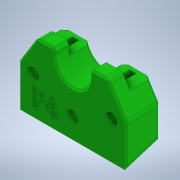
# Autodesk Inventor part: Y-Rod Holder
Saved by Autodesk Inventor 2020 (Build 240168000, 168)
## iProperties
Created: 2019-06-18
Part Number: Y-Rod Holder
Material: ABS Plastic
Document SubType Name: Modeling
Designer: pepd9
Density: 1.06 g/cm^3
Appearance: Dark Green
Author: pepd9
Autodesk Inventor part; units mm, degrees
ref_plane "YZ Plane" through (0, 0, 0) normal (1, 0, 0) x (0, 1, 0)
ref_plane "XZ Plane" through (0, 0, 0) normal (0, 1, 0) x (-1, 0, 0)
ref_plane "XY Plane" through (0, 0, 0) normal (0, 0, 1) x (1, 0, 0)
sketch "Sketch1" plane through (0, 0, 0) normal (0, 0, 1) x (1, 0, 0)
  circle A0 centre (0, 0) radius 5
  line L0 (-8, 0) -> (8, 0)
  line L1 (8, 0) -> (8, -12)
  line L2 (8, -12) -> (-8, -12)
  line L3 (-8, -12) -> (-8, 0)
  point P0 (5, 0)
  point P1 (-5, 0)
  dimension "d0" = 10
  dimension "d1" = 8
  dimension "d2" = 8
  dimension "d3" = 12
  constraints: 8 end point, 2 parallel, 1 centre point, 1 coincident, 1 horizontal, 1 perpendicular
  measures "d0" diameter of A0
  measures "d1" distance from line of L1 point (0, 0)
  measures "d2" distance of point (0, 0) L0.start
  measures "d3" distance from line of point (0, 0) L2
extrude "Extrusion1" add sketch "Sketch1" along normal blind 6 contours L0 L1 L2 L3 A0
sketch "Sketch2" plane through (0, 0, 6) normal (0, 0, 1) x (1, 0, 0)
  circle A0 centre (0, 0) radius 5 projected
  line L0 (-15, -18) -> (15, -18)
  line L1 (15, -18) -> (15, 2)
  line L2 (15, 2) -> (-15, 2)
  line L3 (-15, 2) -> (-15, -18)
  point P0 (0, 0)
  point P1 (4.5826, 2)
  point P2 (-4.5826, 2)
  dimension "d6" = 2
  dimension "d7" = 20
  dimension "d8" = 30
  dimension "d9" = 15
  constraints: 8 end point, 2 parallel, 1 horizontal, 1 perpendicular
  measures "d6" distance from line of L2 point (0, 0)
  measures "d7" distance between parallel lines of L2 L0
  measures "d8" distance of L1.end L2.end
  measures "d9" distance from line of L1 point (0, 0)
extrude "Extrusion2" add sketch "Sketch2" against normal blind 10 contours A0 L2 L1 L0 L3
chamfer "Chamfer1" distance 1 angle 45 2 edges at (-4.5826, 2, 1) (4.5826, 2, 1)
sketch "Sketch3" plane through (-15, 2, 6) normal (0, 1, 0) x (1, 0, 0)
  line L0 (9.1674, 5.5) -> (7.3674, 5.5)
  line L1 (7.3674, 5.5) -> (7.3674, 9)
  line L2 (7.3674, 9) -> (9.1674, 9)
  line L3 (9.1674, 9) -> (9.1674, 5.5)
  line L4 (9.1674, 5.5) -> (7.3674, 9) construction
  line L5 (7.3674, 5.5) -> (9.1674, 9) construction
  line L6 (0, 10) -> (9.4174, 10) projected
  line L7 (9.4174, 10) -> (9.4174, 0) projected
  point P0 (15, 6)
  point P1 (8.2674, 7.25)
  dimension "d15" = 1.8
  dimension "d16" = 3.5
  dimension "d17" = 1
  dimension "d18" = 0.25
  constraints: 12 end point, 2 midpoint, 2 parallel, 1 horizontal, 1 perpendicular
  measures "d15" distance of L1.end L2.end
  measures "d16" distance of L0.end L1.end
  measures "d17" distance between parallel lines of L6 L2
  measures "d18" distance between parallel lines of L3 L7
ref_plane "Work Plane1" through (0, 0, -3) normal (0, 0, -1) x (-1, 0, 0)
sketch "Sketch4" plane through (0, 0, -3) normal (0, 0, -1) x (-1, 0, 0)
  line L0 (15, 2) -> (5.5826, 2) projected
  line L1 (5.8326, 2) -> (7.2498, -1.8938)
  arc A0 (4.3864, -5.3999) -> (7.3385, -2.9339) centre (4.3864, -2.3999) ccw
  line L2 (4.3864, -5.3999) -> (0, -5.3999)
  arc A1 (-4.8889, 1.0481) -> (4.8889, 1.0481) centre (0, 0) ccw projected
  line L3 (0, 0) -> (0, 3.0326)
  line L4 (-5.8326, 2) -> (-7.2498, -1.8938)
  arc A2 (-7.3385, -2.9339) -> (-4.3864, -5.3999) centre (-4.3864, -2.3999) ccw
  line L5 (-4.3864, -5.3999) -> (0, -5.3999)
  arc A3 (7.3385, -2.9339) -> (7.2498, -1.8938) centre (5.3704, -2.5779) ccw
  arc A4 (-7.2498, -1.8938) -> (-7.3385, -2.9339) centre (-5.3704, -2.5779) ccw
  point P0 (0, 0)
  point P1 (7.3831, -2.2602)
  point P2 (-7.3831, -2.2602)
  point P3 (7.3831, -2.2602)
  point P4 (5.8326, 2)
  point P5 (-7.3831, -2.2602)
  dimension "d20" = 6
  dimension "d24" = 70
  dimension "d25" = 2
  constraints: 12 point on circle, 10 end point, 5 symmetric about line, 5 tangent, 4 centre point, 4 point on line, 1 equal radius, 1 horizontal, 1 vertical, 1 other
  measures "d20" diameter of A0
  measures "d24" angle of L0 L1
  measures "d25" radius of A3
sweep "Sweep1" cut profiles "Sketch3" path "Sketch4" path curves L1 A3 A0 L2 L5 A2 A4 L4
sketch "Sketch5" plane through (0, 0, 6) normal (0, 0, 1) x (1, 0, 0)
  line L0 (5.8326, 2) -> (7.6326, 2) projected
  line L1 (7.2498, -1.8938) -> (5.8326, 2) projected
  arc A0 (7.3385, -2.9339) -> (7.2498, -1.8938) centre (5.3704, -2.5779) ccw projected
  arc A1 (4.3864, -5.3999) -> (7.3385, -2.9339) centre (4.3864, -2.3999) ccw projected
  line L2 (-4.3864, -5.3999) -> (4.3864, -5.3999) projected
  arc A2 (-7.3385, -2.9339) -> (-4.3864, -5.3999) centre (-4.3864, -2.3999) ccw projected
  arc A3 (-7.2498, -1.8938) -> (-7.3385, -2.9339) centre (-5.3704, -2.5779) ccw projected
  line L3 (-5.8326, 2) -> (-7.2498, -1.8938) projected
  line L4 (-7.6326, 2) -> (-5.8326, 2) projected
  line L5 (-7.6326, 2) -> (-9.0498, -1.8938) projected
  arc A4 (-9.0498, -1.8938) -> (-8.8933, -3.8408) centre (-5.3704, -2.5779) ccw projected
  arc A5 (-8.8933, -3.8408) -> (-3.7708, -7.0913) centre (-4.3864, -2.3999) ccw projected
  line L6 (-3.7708, -7.0913) -> (5.002, -7.0913) projected
  arc A6 (5.002, -7.0913) -> (9.1125, -2.6292) centre (4.3864, -2.3999) ccw projected
  arc A7 (9.1125, -2.6292) -> (8.6287, -0.7368) centre (5.3704, -2.5779) ccw projected
  line L7 (8.6287, -0.7368) -> (7.6326, 2) projected
  line L8 (-9.4123, -4.3413) -> (-7.8246, -7.0913)
  line L9 (-7.8246, -7.0913) -> (-9.4123, -9.8413)
  line L10 (-9.4123, -9.8413) -> (-12.5877, -9.8413)
  line L11 (-12.5877, -9.8413) -> (-14.1754, -7.0913)
  line L12 (-14.1754, -7.0913) -> (-12.5877, -4.3413)
  line L13 (-12.5877, -4.3413) -> (-9.4123, -4.3413)
  line L14 (1.5877, -9.25) -> (3.1754, -12)
  line L15 (3.1754, -12) -> (1.5877, -14.75)
  line L16 (1.5877, -14.75) -> (-1.5877, -14.75)
  line L17 (-1.5877, -14.75) -> (-3.1754, -12)
  line L18 (-3.1754, -12) -> (-1.5877, -9.25)
  line L19 (-1.5877, -9.25) -> (1.5877, -9.25)
  line L20 (0, 0) -> (0, 7.1717)
  line L21 (9.4123, -4.3413) -> (7.8246, -7.0913)
  line L22 (7.8246, -7.0913) -> (9.4123, -9.8413)
  line L23 (9.4123, -9.8413) -> (12.5877, -9.8413)
  line L24 (12.5877, -9.8413) -> (14.1754, -7.0913)
  line L25 (14.1754, -7.0913) -> (12.5877, -4.3413)
  line L26 (12.5877, -4.3413) -> (9.4123, -4.3413)
  point P0 (0, -12)
  point P1 (-11, -7.0913)
  point P2 (-11, -7.0913)
  point P3 (0, -12)
  point P4 (11, -7.0913)
  dimension "d28" = 5.5
  dimension "d29" = 5.5
  dimension "d31" = 11
  dimension "d32" = 12
  constraints: 38 end point, 7 symmetric about line, 2 coincident, 1 vertical, 1 vertical alignment, 26 other
  measures "d28" distance between parallel lines of L13 L10
  measures "d29" distance between parallel lines of L16 L19
  measures "d31" horizontal distance of L20.start point (-11, -7.091)
  measures "d32" distance of L20.start point (0, -12)
sketch "Sketch6" plane through (0, 0, -4) normal (0, 0, -1) x (-1, 0, 0)
  line L0 (-9.4123, -4.3413) -> (-7.8246, -7.0913)
  line L1 (-7.8246, -7.0913) -> (-9.4123, -9.8413)
  line L2 (-9.4123, -9.8413) -> (-12.5877, -9.8413)
  line L3 (-12.5877, -9.8413) -> (-14.1754, -7.0913)
  line L4 (-14.1754, -7.0913) -> (-12.5877, -4.3413)
  line L5 (-12.5877, -4.3413) -> (-9.4123, -4.3413)
  line L6 (1.5877, -9.25) -> (3.1754, -12)
  line L7 (3.1754, -12) -> (1.5877, -14.75)
  line L8 (1.5877, -14.75) -> (-1.5877, -14.75)
  line L9 (-1.5877, -14.75) -> (-3.1754, -12)
  line L10 (-3.1754, -12) -> (-1.5877, -9.25)
  line L11 (-1.5877, -9.25) -> (1.5877, -9.25)
  line L12 (12.5877, -4.3413) -> (14.1754, -7.0913)
  line L13 (14.1754, -7.0913) -> (12.5877, -9.8413)
  line L14 (12.5877, -9.8413) -> (9.4123, -9.8413)
  line L15 (9.4123, -9.8413) -> (7.8246, -7.0913)
  line L16 (7.8246, -7.0913) -> (9.4123, -4.3413)
  line L17 (9.4123, -4.3413) -> (12.5877, -4.3413)
  point P0 (0, 0)
  point P1 (-11, -7.0913)
  point P2 (0, -12)
  point P3 (11, -7.0913)
  point P4 (-11, -7.0913)
  point P5 (0, -12)
  point P6 (11, -7.0913)
  point P7 (11, -4.3413)
  dimension "d33" = 5.5
  dimension "d34" = 5.5
  dimension "d35" = 5.5
  constraints: 36 end point, 3 coincident, 1 midpoint, 1 point on line, 39 other
  measures "d33" distance between parallel lines of L5 L2
  measures "d34" distance between parallel lines of L11 L8
  measures "d35" distance between parallel lines of L17 L14
extrude "Extrusion3" cut sketch "Sketch6" against normal blind 5
hole "Hole1" at (0, -12, 6) at (-11, -7.0913, 6) at (11, -7.0913, 6) direction (0, 0, -1) diameter 3.2 end through all
chamfer "Chamfer2" distance 8 distance2 5 1 edges at (-15, 2, 1) measured on face at (-15, 1.5, 1)
chamfer "Chamfer3" distance 5 distance2 8 1 edges at (15, 2, 1) measured on face at (14.5, 2, 1)
chamfer "Chamfer4" distance 0.25 distance2 4.5 1 edges at (11, -4.3413, -4) measured on face at (11, -3.8413, -4)
chamfer "Chamfer5" distance 0.25 distance2 4.5 2 edges at (12.5155, -4.2163, -4) (13.3816, -5.7163, -4) measured on face at (12.9486, -3.9663, -4) measured on face at (13.8146, -5.4663, -4)
chamfer "Chamfer6" distance 0.25 distance2 4.5 2 edges at (14.2476, -6.9663, -4) (13.3816, -8.4663, -4) measured on face at (14.6806, -7.2163, -4) measured on face at (13.8146, -8.7163, -4)
chamfer "Chamfer7" distance 0.25 distance2 4.5 2 edges at (12.7321, -9.8413, -4) (11, -9.8413, -4) measured on face at (11, -10.3413, -4) measured on face at (12.7321, -10.3413, -4)
chamfer "Chamfer8" distance 0.25 distance2 4.5 2 edges at (9.4845, -9.9663, -4) (8.6184, -8.4663, -4) measured on face at (9.0514, -10.2163, -4) measured on face at (8.1854, -8.7163, -4)
chamfer "Chamfer9" distance 0.25 distance2 4.5 3 edges at (7.7524, -7.2163, -4) (8.6184, -5.7163, -4) (9.4845, -4.2163, -4) measured on face at (7.3194, -6.9663, -4) measured on face at (9.0514, -3.9663, -4) measured on face at (8.1854, -5.4663, -4)
chamfer "Chamfer10" distance 0.25 distance2 4.5 1 edges at (0, -9.25, -4) measured on face at (0, -8.75, -4)
chamfer "Chamfer11" distance 0.25 distance2 4.5 2 edges at (1.5155, -9.125, -4) (2.3816, -10.625, -4) measured on face at (1.9486, -8.875, -4) measured on face at (2.8146, -10.375, -4)
chamfer "Chamfer12" distance 0.25 distance2 4.5 2 edges at (3.2476, -11.875, -4) (2.3816, -13.375, -4) measured on face at (2.8146, -13.625, -4) measured on face at (3.6806, -12.125, -4)
chamfer "Chamfer13" distance 0.25 distance2 4.5 2 edges at (1.7321, -14.75, -4) (0, -14.75, -4) measured on face at (0, -15.25, -4) measured on face at (1.7321, -15.25, -4)
chamfer "Chamfer14" distance 0.25 distance2 4.5 2 edges at (-1.5155, -14.875, -4) (-2.3816, -13.375, -4) measured on face at (-2.8146, -13.625, -4) measured on face at (-1.9486, -15.125, -4)
chamfer "Chamfer15" distance 0.25 distance2 4.5 3 edges at (-3.2476, -12.125, -4) (-2.3816, -10.625, -4) (-1.5155, -9.125, -4) measured on face at (-1.9486, -8.875, -4) measured on face at (-3.6806, -11.875, -4) measured on face at (-2.8146, -10.375, -4)
chamfer "Chamfer16" distance 0.25 distance2 4.5 1 edges at (-8.6184, -5.7163, -4) measured on face at (-8.1854, -5.4663, -4)
chamfer "Chamfer17" distance 0.25 distance2 4.5 2 edges at (-7.7524, -6.9663, -4) (-8.6184, -8.4663, -4) measured on face at (-7.3194, -7.2163, -4) measured on face at (-8.1854, -8.7163, -4)
chamfer "Chamfer18" distance 0.25 distance2 4.5 2 edges at (-9.2679, -9.8413, -4) (-11, -9.8413, -4) measured on face at (-11, -10.3413, -4) measured on face at (-9.2679, -10.3413, -4)
chamfer "Chamfer19" distance 0.25 distance2 4.5 2 edges at (-12.5156, -9.9663, -4) (-13.3816, -8.4663, -4) measured on face at (-13.8146, -8.7163, -4) measured on face at (-12.9486, -10.2163, -4)
chamfer "Chamfer20" distance 0.25 distance2 4.5 2 edges at (-14.2476, -7.2163, -4) (-13.3816, -5.7163, -4) measured on face at (-14.6806, -6.9663, -4) measured on face at (-13.8146, -5.4663, -4)
chamfer "Chamfer21" distance 0.25 distance2 4.5 3 edges at (-12.732, -4.3413, -4) (-11, -4.3413, -4) (-9.2679, -4.3413, -4) measured on face at (-11, -3.8413, -4) measured on face at (-9.2679, -3.8413, -4) measured on face at (-12.732, -3.8413, -4)
chamfer "Chamfer22" distance 2.5 distance2 8 1 edges at (0, -18, -4) measured on face at (0, -17.5, -4)
chamfer "Chamfer23" distance 0.5 angle 45 10 edges at (-15, -12, 6) (0, -18, 6) (15, -12, 6) (12.5, -2, 6) (7.7913, 2, 6) (5.2357, 1.524, 6) (0, -5, 6) (-5.2357, 1.524, 6) (-7.7913, 2, 6) (-12.5, -2, 6)
chamfer "Chamfer24" distance 1 angle 45 8 edges at (0, -15.5, -4) (15, -10.75, -4) (-15, -10.75, -4) (-12.5, -2, -4) (-7.7913, 2, -4) (7.7913, 2, -4) (12.5, -2, -4) (0, -5, -4)
fillet "Fillet1" radius 2 6 edges at (-15, -6, 1.25) (15, -6, 1.25) (15, -16.9062, 0.5) (-15, -16.9062, 0.5) (-10, 2, 1.25) (10, 2, 1.25)
sketch "Sketch7" plane through (0, 0, 6) normal (0, 0, 1) x (1, 0, 0)
  line L0 (-11.0548, -9.9411) -> (-3.6947, -9.9411) construction
  line L1 (-3.6947, -9.9411) -> (-3.6947, -14.9411) construction
  line L2 (-3.6947, -14.9411) -> (-11.0548, -14.9411) construction
  line L3 (-11.0548, -14.9411) -> (-11.0548, -9.9411) construction
  line L4 (-10.7864, -14.9411) -> (-10.7864, -9.9411)
  line L5 (-10.7864, -9.9411) -> (-8.8363, -9.9411)
  spline S0 degree 2 poles (-8.8363, -9.9411) (-8.1577, -9.9411) (-7.453, -10.5339) (-7.3487, -11.1715) knots 0 0 0 1 2 2 2
  spline S1 degree 2 poles (-7.3487, -11.1715) (-7.3188, -11.3803) (-7.3114, -11.5257) (-7.3114, -11.5817) knots 0 0 0 1 2 2 2
  spline S2 degree 2 poles (-7.3114, -11.5817) (-7.3114, -12.2864) (-8.1838, -13.0768) (-8.9631, -13.0768) knots 0 0 0 1 2 2 2
  line L6 (-8.9631, -13.0768) -> (-9.3583, -13.0768)
  line L7 (-9.3583, -13.0768) -> (-9.3583, -14.9411)
  line L8 (-9.3583, -14.9411) -> (-10.7864, -14.9411)
  spline S3 degree 2 poles (-9.1458, -12.0254) (-9.0414, -12.0254) (-8.8177, -11.8501) (-8.7804, -11.6712) knots 0 0 0 1 2 2 2
  spline S4 degree 2 poles (-8.7804, -11.6712) (-8.7618, -11.5779) (-8.7618, -11.4959) knots 0 0 0 1 1 1
  spline S5 degree 2 poles (-8.7618, -11.4959) (-8.7618, -11.2647) (-8.978, -11) (-9.1309, -11) knots 0 0 0 1 2 2 2
  line L9 (-9.1309, -11) -> (-9.3583, -11)
  line L10 (-9.3583, -11) -> (-9.3583, -12.0254)
  line L11 (-9.3583, -12.0254) -> (-9.1458, -12.0254)
  line L12 (-7.2629, -13.9419) -> (-7.2629, -12.9016)
  line L13 (-7.2629, -12.9016) -> (-5.7305, -9.9411)
  line L14 (-5.7305, -9.9411) -> (-4.2465, -9.9411)
  line L15 (-4.2465, -9.9411) -> (-4.2465, -12.8904)
  line L16 (-4.2465, -12.8904) -> (-3.814, -12.8904)
  line L17 (-3.814, -12.8904) -> (-3.814, -13.9419)
  line L18 (-3.814, -13.9419) -> (-4.2465, -13.9419)
  line L19 (-4.2465, -13.9419) -> (-4.2465, -14.9411)
  line L20 (-4.2465, -14.9411) -> (-5.6, -14.9411)
  line L21 (-5.6, -14.9411) -> (-5.6, -13.9456)
  spline S6 degree 2 poles (-5.6, -13.9456) (-5.6261, -13.9419) (-5.9132, -13.9419) (-6.0548, -13.9419) knots 0 0 0 1 2 2 2
  spline S7 degree 2 poles (-6.0548, -13.9419) (-6.4314, -13.9419) (-6.9609, -13.9419) (-7.2629, -13.9419) knots 0 0 0 1 2 2 2
  line L22 (-5.5515, -12.8904) -> (-5.5515, -11.4363)
  line L23 (-5.5515, -11.4363) -> (-6.1704, -12.8904)
  line L24 (-6.1704, -12.8904) -> (-5.5515, -12.8904)
  point P0 (0, 0)
  constraints: 2 other
extrude "Extrusion4" cut sketch "Sketch7" against normal blind 0.4
sketch "Sketch8" plane through (0, 0, -4) normal (0, 0, -1) x (-1, 0, 0)
  line L0 (-15.8889, 5.7787) -> (16.1256, 5.7787)
  line L1 (16.1256, 5.7787) -> (16.1256, -1.5)
  line L2 (16.1256, -1.5) -> (-15.8889, -1.5)
  line L3 (-15.8889, -1.5) -> (-15.8889, 5.7787)
  point P0 (0, 0)
  dimension "d117" = 1.5
  constraints: 8 end point, 2 parallel, 1 horizontal, 1 perpendicular
  measures "d117" distance from line of point (0, 0) L2
extrude "Extrusion5" cut sketch "Sketch8" against normal blind 6
body "Solid1"
